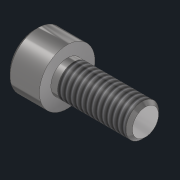
# Autodesk Inventor part: CB5-12
Saved by Autodesk Inventor 2022 (Build 260153000, 153)
## iProperties
Category: PARTsolutions
Company: MISUMI
Created: 2016-12-21
Part Number: CB5-12
Catalog Web Link: www.cadenas.de
Description: CB-Hexagon Socket Head Cap Screws
Vendor: MISUMI
Document SubType Name: Modeling
Designer: psAdmin
Manufacturer: MISUMI
Mass: 3.74826 g
Surface Area: 4.57615 cm^2
Volume: 0.477486 cm^3
Density: 7.85 g/cm^3
Material: 鋼、炭素鋼
Appearance: 半つや出し
PSOL_IDENT_0: {$CADENAS_DATA\23d-libs\misumi\metric\27_screws_nuts\cb_fa.prj},151 {VTYP=3D},{NB=CB5-12},{LINA=CB5-
PSOL_IDENT_1: 12},{NN=CB},{DATE=17.06.2016 05:50:53},{GEOMDATE=17.02.2014 00:00:00},{VERSION=},{LINEID=40},{LINESU
PSOL_IDENT_2: BID=-1},{WBVAR=L}  {NB=CB5-12},{LINA=CB5-12},{KT=DUMMY},{PN=CB5-12},{MAT=4137 Steel},{HARD=38~43HRC}
PSOL_IDENT_3: ,{ST=Black Oxide},{M=5},{L=12},{LL=Full Thread},{L1=22},{TYPE=CB},{M1=5.000},{L0=5,6,8,10,12,14,15,1
PSOL_IDENT_4: 6,18,20,22,25,30,35,40,45,50,55,60,65,70,75,80},{NDM=5},{KDM=4.017064},{MP=5x0.8},{P=0.8},{A=8.5},{E=
PSOL_IDENT_5: 5.0},{B=4.0},{V=0.5}
NN: CB
NT: Hexagon Socket Head Cap Screws
NB: CB5-12
NBSYN: $PN.
LINA: CB5-12
PN: CB5-12
MAT: 4137 Steel
HARD: 38~43HRC
ST: Black Oxide
M: 5
L: 12
LL: Full Thread
MP: 5x0.8
A: 8.5
E: 5.0
B: 4.0
SUPPLIER: MISUMI
ARTICLENO: CB5-12
BOMINFO: CB5-12
CREATOR: CADENAS GmbH
購入先: ミスミ
在庫数: 0.0
Title: CB5-12
Author: Cadenas PARTsolutions
Comments: Hexagon Socket Head Cap Screws
Autodesk Inventor part; units mm, degrees
sketch "Sketch_1" plane through (0, 0, 0) normal (0, 0, 1) x (1, 0, 0)
  line L0 (12, 0) -> (-5, 0)
  line L1 (-5, 0) -> (-5, 3.75)
  line L2 (-5, 3.75) -> (-4.5, 4.25)
  line L3 (-4.5, 4.25) -> (0, 4.25)
  line L4 (0, 4.25) -> (0, 2.5)
  line L5 (0, 2.5) -> (11.5095, 2.5)
  line L6 (11.5095, 2.5) -> (12, 2.0095)
  line L7 (12, 2.0095) -> (12, 0)
  line L8 (12, 0) -> (-5, 0)
  constraints: 18 end point
revolve "Revolution1" add sketch "Sketch_1" angle 360 about axis through (12, 0, 0) along (1, 0, 0)
thread "Thread1" size "M5x0.8" class "6g" standard "ISO Metric profile" length 10.5095
sketch "Sketch2" plane through (-5, 0, 0) normal (-1, 0, 0) x (0, 0, 1)
  point P0 (0, 0)
hole "Hole1" at (-5, 0, 0) direction (1, 0, 0) diameter 4 depth 2.5 tip angle 150
sketch "Sketch_3" plane through (-5, 0, 0) normal (1, 0, 0) x (0, 0, -1)
  line L0 (-2, 1.1547) -> (-2, -1.1547)
  line L1 (-2, -1.1547) -> (0, -2.3094)
  line L2 (0, -2.3094) -> (2, -1.1547)
  line L3 (2, -1.1547) -> (2, 1.1547)
  line L4 (2, 1.1547) -> (0, 2.3094)
  line L5 (0, 2.3094) -> (-2, 1.1547)
  constraints: 12 end point
extrude "Extrusion1" cut sketch "Sketch_3" along normal blind 2.5
ref_plane "bolt_to_nut_XY" through (12, 0, 0) normal (1, 0, 0) x (0, 0, -1)
ref_plane "bolt_to_nut_YZ" through (12, 0, 0) normal (0, 0, -1) x (0, 1, 0)
ref_plane "bolt_to_nut_ZX" through (12, 0, 0) normal (0, 1, 0) x (1, 0, 0)
ref_plane "screw1_XY" through (0, 0, 0) normal (1, 0, 0) x (0, 0, -1)
ref_plane "screw1_YZ" through (0, 0, 0) normal (0, 0, -1) x (0, 1, 0)
ref_plane "screw1_ZX" through (0, 0, 0) normal (0, 1, 0) x (1, 0, 0)
body "Solid1"
